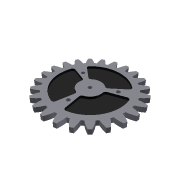
# Autodesk Inventor part: 平歯車1
Saved by Autodesk Inventor 2011 SP1 (Build 150282100, 282)
## iProperties
Created: 2012-11-22
Part Number: 平歯車1
Material: Steel
Document SubType Name: Modeling
Designer: arihon
Categories: <?xml version="1.0" encoding="UTF-16"?> <MemberInstance><Categories><FamilyTemplate><FamilyTemplateParameter ValueType="xs:double" Id="1" ObjectReferenceKey="da_z" ObjectType="kUserParameterObject"/><FamilyTemplateParameter ValueType="xs:double" Id="2" ObjectReferenceKey="da_b" ObjectType="kUserParameterObject"/><FamilyTemplateParameter ValueType="xs:double" Id="3" ObjectReferenceKey="da_beta" ObjectType="kUserParameterObject"/><FamilyTemplateParameter ValueType="xs:double" Id="4" ObjectReferenceKey="da_da" ObjectType="kUserParameterObject"/><FamilyTemplateParameter ValueType="xs:double" Id="5" ObjectReferenceKey="da_aw" ObjectType="kUserParameterObject"/><FamilyTemplateParameter ValueType="xs:string" Id="6" ObjectReferenceKey="EAIAABAAAACIAQAAAAAAAIAAAAAAAAAA" ObjectType="83910656" SubObjectId="SurfaceGeometry"/></FamilyTemplate><ParamToTemplateMap><ParamToTemplate CategoryParameter="//CategoryParameter[@InternalName='046C89C9-8512-4d59-83FE-43B91F4F132A']" TemplateParameter="1"/><ParamToTemplate CategoryParameter="//CategoryParameter[@InternalName='2552DF32-E462-4b46-AEBF-C6C7768E72AC']" TemplateParameter="2"/><ParamToTemplate CategoryParameter="//CategoryParameter[@InternalName='C9EE641D-15FC-4fae-A226-E94C4372FDD7']" TemplateParameter="3"/><ParamToTemplate><ParamToTemplate CategoryParameter="//CategoryParameter[@InternalName='00B6519A-459B-49c7-AD84-2E56D39A5744']" ConstantValue="0.000000"/></ParamToTemplate><ParamToTemplate><ParamToTemplate CategoryParameter="//CategoryParameter[@InternalName='04B31F0E-C7A6-4894-AA32-9629BEFACF47']" ConstantValue="1.000000"/></ParamToTemplate><ParamToTemplate><ParamToTemplate CategoryParameter="//CategoryParameter[@InternalName='43CBEC2E-7847-49e7-A936-2F7889FCB2D9']" ConstantValue="0.250000"/></ParamToTemplate><ParamToTemplate><ParamToTemplate CategoryParameter="//CategoryParameter[@InternalName='B1EFC894-105D-4ebd-86BF-FA20ED196853']" ConstantValue="0.350000"/></ParamToTemplate><ParamToTemplate><ParamToTemplate CategoryParameter="//CategoryParameter[@InternalName='51175063-3D10-4879-93E8-6246FE8B403D']" ConstantValue="2060000000.000000"/></ParamToTemplate><ParamToTemplate><ParamToTemplate CategoryParameter="//CategoryParameter[@InternalName='A3A52E27-4454-46a9-B0BD-C932399B70AF']" ConstantValue="0.300000"/></ParamToTemplate><ParamToTemplate><ParamToTemplate CategoryParameter="//CategoryParameter[@InternalName='91B76062-C214-41d9-B1B9-14D2AB99603D']" ConstantValue="0.300000"/></ParamToTemplate><ParamToTemplate><ParamToTemplate CategoryParameter="//CategoryParameter[@InternalName='374E806E-8B8A-4dda-A9AA-1039D6500AD2']" ConstantValue="3.333333"/></ParamToTemplate><ParamToTemplate><ParamToTemplate CategoryParameter="//CategoryParameter[@InternalName='2D373A89-B862-43d6-8D0B-0CBF12AB9F6C']" ConstantValue="0.349066"/></ParamToTemplate><ParamToTemplate CategoryParameter="//CategoryParameter[@InternalName='37777632-D6A2-4fac-9D53-DB8ACD95C989']" TemplateParameter="4"/><ParamToTemplate CategoryParameter="//CategoryParameter[@InternalName='FD1017F1-B727-4f7e-9707-0F86F1FF9423']" TemplateParameter="5"/><ParamToTemplate><ParamToTemplate CategoryParameter="//CategoryParameter[@InternalName='9E1B4470-B2D3-4ff1-B813-535BB4CDF51A']" ConstantValue="3520000.000000"/></ParamToTemplate><ParamToTemplate><ParamToTemplate CategoryParameter="//CategoryParameter[@InternalName='F8452263-BFF6-458c-9FB1-07C4B99E95CD']" ConstantValue="11400000.000000"/></ParamToTemplate><ParamToTemplate><ParamToTemplate CategoryParameter="//CategoryParameter[@InternalName='3E3BB259-FD49-497f-8171-6EBC954A3479']" ConstantValue="2.000000"/></ParamToTemplate><ParamToTemplate CategoryParameter="//CategoryParameter[@InternalName='27C3BAF2-7550-4e4b-AE2C-0DB134B7D9B7']" TemplateParameter="6"/></ParamToTemplateMap><Category DisplayName="Gear" InternalName="DC85795E-93AB-48d5-8EEE-5A27447B64BD" Mnemonic="Gear"><CategoryParameter DisplayName="z" InternalName="046C89C9-8512-4d59-83FE-43B91F4F132A" Mnemonic="z"/><CategoryParameter DisplayName="b" InternalName="2552DF32-E462-4b46-AEBF-C6C7768E72AC" Mnemonic="b"/><CategoryParameter DisplayName="||b|" InternalName="C9EE641D-15FC-4fae-A226-E94C4372FDD7" Mnemonic="beta"/><CategoryParameter DisplayName="x" InternalName="00B6519A-459B-49c7-AD84-2E56D39A5744" Mnemonic="x"/><CategoryParameter DisplayName="a*" InternalName="04B31F0E-C7A6-4894-AA32-9629BEFACF47" Mnemonic="a"/><CategoryParameter DisplayName="c*" InternalName="43CBEC2E-7847-49e7-A936-2F7889FCB2D9" Mnemonic="c"/><CategoryParameter DisplayName="r|.f|*" InternalName="B1EFC894-105D-4ebd-86BF-FA20ED196853" Mnemonic="rf"/><CategoryParameter DisplayName="E" InternalName="51175063-3D10-4879-93E8-6246FE8B403D" Mnemonic="E"/><CategoryParameter DisplayName="||m|" InternalName="A3A52E27-4454-46a9-B0BD-C932399B70AF" Mnemonic="mi"/><Category DisplayName="SpurGear" InternalName="26C5A22E-A91E-4dfd-A3B3-23CCAFAE1764" Mnemonic="SpurGear"><CategoryParameter DisplayName="m" InternalName="91B76062-C214-41d9-B1B9-14D2AB99603D" Mnemonic="m"/><CategoryParameter DisplayName="P" InternalName="374E806E-8B8A-4dda-A9AA-1039D6500AD2" Mnemonic="PP"/><CategoryParameter DisplayName="||a|" InternalName="2D373A89-B862-43d6-8D0B-0CBF12AB9F6C" Mnemonic="alpha"/><CategoryParameter DisplayName="d|.a|" InternalName="37777632-D6A2-4fac-9D53-DB8ACD95C989" Mnemonic="da"/><CategoryParameter DisplayName="a|.w|" InternalName="FD1017F1-B727-4f7e-9707-0F86F1FF9423" Mnemonic="aw"/><CategoryParameter DisplayName="||s||.Flim|" InternalName="9E1B4470-B2D3-4ff1-B813-535BB4CDF51A" Mnemonic="sFlim"/><CategoryParameter DisplayName="||s||.Hlim|" InternalName="F8452263-BFF6-458c-9FB1-07C4B99E95CD" Mnemonic="sHlim"/><CategoryParameter DisplayName="種類" InternalName="3E3BB259-FD49-497f-8171-6EBC954A3479" Mnemonic="type"/><CategoryParameter DisplayName="PitchDiameter" InternalName="27C3BAF2-7550-4e4b-AE2C-0DB134B7D9B7" Mnemonic="IDS_PITCHDIAM"/></Category></Category></Categories></MemberInstance>
Density: 1 g/cm^3
CustomPartVersion: 1
Author: arihon
Autodesk Inventor part; units mm, degrees
ref_plane "YZ Plane" through (0, 0, 0) normal (1, 0, 0) x (0, 1, 0)
ref_plane "XZ Plane" through (0, 0, 0) normal (0, 1, 0) x (-1, 0, 0)
ref_plane "XY Plane" through (0, 0, 0) normal (0, 0, 1) x (1, 0, 0)
sketch "Sketch1" plane through (0, 0, 0) normal (0, 0, 1) x (1, 0, 0)
  circle A0 centre (0, 0) radius 38.9632
  dimension "d0" = 77.9263
  constraints: 1 centre point
  measures "d0" diameter of A0
extrude "Extrusion1" add sketch "Sketch1" along normal blind 5
ref_plane "Work Plane2" through (0, 0, 2.5) normal (0, 0, 1) x (1, 0, 0)
sketch "Sketch2" plane through (0, 0, 0) normal (0, 0, -1) x (-1, 0, 0)
  circle A0 centre (0, 0) radius 38.9632 projected
  circle A1 centre (0, 0) radius 36.3636
  dimension "d3" = 72.7273
  constraints: 1 centre point, 1 coincident
  measures "d3" diameter of A1
surface extrude "ピッチ円直径" sketch "Sketch2" against normal through all shown no curves A1
ref_plane "Work Plane8" through (0, 0, 0) normal (0.9914449, 0.1305262, 0) x (0, 0, 1)
ref_plane "Work Plane9" through (0, 0, 0) normal (1, 0, 0) x (0, 1, 0)
spur gear teeth "平歯車" teeth 24 pitch diameter 72 tip diameter 77.9263 root diameter 64.5 face width 5 start plane through (0, 0, 0) normal (0, 0, -1) x (-1, 0, 0)
sketch "スケッチ3" plane through (0, 0, 5) normal (0, 0, 1) x (1, 0, 0)
  arc A0 (-8.8476, 37.9453) -> (-11.3104, 37.2854) centre (0, 0) ccw projected
  arc A1 (-21.0662, 17.6767) -> (21.0662, 17.6767) centre (0, 0) ccw
  arc A2 (0, 10) -> (-7.6604, 6.4279) centre (0, 0) ccw
  line L0 (0, 0) -> (-7.6604, 6.4279)
  line L1 (0, 0) -> (7.6604, 6.4279)
  line L2 (0, 0) -> (0, 27.5)
  line L3 (7.6604, 6.4279) -> (21.0662, 17.6767)
  line L4 (-7.6604, 6.4279) -> (-21.0662, 17.6767)
  arc A3 (0, 27.5) -> (-21.0662, 17.6767) centre (0, 0) ccw
  arc A4 (21.0662, 17.6767) -> (0, 27.5) centre (0, 0) ccw
  arc A5 (7.6604, 6.4279) -> (0, 10) centre (0, 0) ccw
  arc A6 (-7.6604, 6.4279) -> (7.6604, 6.4279) centre (0, 0) ccw
  dimension "d49" = 55
  dimension "d50" = 20
  dimension "d51" = 100
  dimension "d52" = 50
  constraints: 12 point on circle, 10 end point, 6 centre point, 3 coincident, 1 point on line, 1 vertical
  measures "d49" diameter of A1
  measures "d50" diameter of A2
  measures "d51" angle of L1 L0
  measures "d52" angle of L1 L2
extrude "押し出し2" cut sketch "スケッチ3" against normal blind 3 contours A3 L2 A2 L4 | L3 A5 L2 A4
fillet "フィレット1" radius 2 4 edges at (-21.0662, 17.6767, 3.5) (-7.6604, 6.4279, 3.5) (7.6604, 6.4279, 3.5) (21.0662, 17.6767, 3.5)
pattern_circular "放射状パターン1" count 3 over 360 about axis through (0, 0, 5) along (0, 0, -1) of "押し出し2", "フィレット1"
sketch "スケッチ5" plane through (0, 0, 5) normal (0, 0, 1) x (1, 0, 0)
  line L0 (19.474, 16.3406) -> (9.064, 7.6056) projected
  arc A0 (20.5752, 33.0876) -> (18.3671, 34.3624) centre (0, 0) ccw projected
  arc A1 (-8.8476, 37.9453) -> (-11.3104, 37.2854) centre (0, 0) ccw projected
  circle A2 centre (0, 0) radius 18.75
  line L1 (0, 0) -> (0, 18.75)
  line L2 (0, 0) -> (16.238, 9.375)
  point P0 (16.238, 9.375)
  point P1 (-16.238, 9.375)
  point P2 (0, -18.75)
  dimension "d71" = 37.5
  dimension "d72" = 60
  dimension "d75" = 360
  constraints: 4 end point, 3 coincident, 2 point on circle, 1 centre point, 1 point on line, 1 vertical, 4 other
  measures "d71" diameter of A2
  measures "d72" angle of L2 L1
hole "Hole2" at (16.238, 9.375, 5) at (-16.238, 9.375, 5) at (0, -18.75, 5) at (0, 0, 5) direction (0, 0, -1) diameter 3.2 depth 8 tip angle 118
sketch "スケッチ6" plane through (0, 0, 5) normal (0, 0, 1) x (1, 0, 0)
  circle A0 centre (0, 0) radius 1.6 projected
  circle A1 centre (0, -18.75) radius 1.6 projected
  circle A2 centre (-16.238, 9.375) radius 1.6 projected
  circle A3 centre (16.238, 9.375) radius 1.6 projected
  line L0 (-23.8883, 8.6946) -> (-11.1186, 4.0468) projected
  arc A4 (-9.8355, 1.8062) -> (-11.1186, 4.0468) centre (-11.8026, 2.1675) ccw projected
  arc A5 (-9.8355, 1.8062) -> (-3.3535, -9.4209) centre (0, 0) ccw projected
  arc A6 (-2.0546, -11.6524) -> (-3.3535, -9.4209) centre (-4.0242, -11.3051) ccw projected
  line L1 (-2.0546, -11.6524) -> (-4.4144, -25.0352) projected
  arc A7 (-6.8847, -26.6243) -> (-4.4144, -25.0352) centre (-6.384, -24.6879) ccw projected
  arc A8 (-26.4996, 7.3498) -> (-6.8847, -26.6243) centre (0, 0) ccw projected
  arc A9 (-23.8883, 8.6946) -> (-26.4996, 7.3498) centre (-24.5724, 6.8153) ccw projected
  line L2 (4.4144, -25.0352) -> (2.0546, -11.6524) projected
  arc A10 (3.3535, -9.4209) -> (2.0546, -11.6524) centre (4.0242, -11.3051) ccw projected
  arc A11 (3.3535, -9.4209) -> (9.8355, 1.8062) centre (0, 0) ccw projected
  arc A12 (11.1186, 4.0468) -> (9.8355, 1.8062) centre (11.8026, 2.1675) ccw projected
  line L3 (11.1186, 4.0468) -> (23.8883, 8.6946) projected
  arc A13 (26.4996, 7.3498) -> (23.8883, 8.6946) centre (24.5724, 6.8153) ccw projected
  arc A14 (6.8847, -26.6243) -> (26.4996, 7.3498) centre (0, 0) ccw projected
  arc A15 (4.4144, -25.0352) -> (6.8847, -26.6243) centre (6.384, -24.6879) ccw projected
  line L4 (19.474, 16.3406) -> (9.064, 7.6056) projected
  arc A16 (6.482, 7.6147) -> (9.064, 7.6056) centre (7.7784, 9.1377) ccw projected
  arc A17 (6.482, 7.6147) -> (-6.482, 7.6147) centre (0, 0) ccw projected
  arc A18 (-9.064, 7.6056) -> (-6.482, 7.6147) centre (-7.7784, 9.1377) ccw projected
  line L5 (-9.064, 7.6056) -> (-19.474, 16.3406) projected
  arc A19 (-19.6149, 19.2745) -> (-19.474, 16.3406) centre (-18.1884, 17.8727) ccw projected
  arc A20 (19.6149, 19.2745) -> (-19.6149, 19.2745) centre (0, 0) ccw projected
  arc A21 (19.474, 16.3406) -> (19.6149, 19.2745) centre (18.1884, 17.8727) ccw projected
  arc A22 (-11.3104, 37.2854) -> (-11.3601, 30.183) centre (15.4473, 33.5469) ccw projected
  arc A23 (-11.3601, 30.183) -> (-13.3098, 29.3754) centre (0, 0) ccw projected
  arc A24 (-13.3098, 29.3754) -> (-18.3671, 34.3624) centre (-34.6442, 12.7984) ccw projected
  arc A25 (-18.3671, 34.3624) -> (-20.5752, 33.0876) centre (0, 0) ccw projected
  arc A26 (-20.5752, 33.0876) -> (-18.7849, 26.2143) centre (6.2384, 36.4019) ccw projected
  arc A27 (-18.7849, 26.2143) -> (-20.4592, 24.9296) centre (0, 0) ccw projected
  arc A28 (-20.4592, 24.9296) -> (-26.6349, 28.4378) centre (-36.7762, 3.3957) ccw projected
  arc A29 (-26.6349, 28.4378) -> (-28.4378, 26.6349) centre (0, 0) ccw projected
  arc A30 (-28.4378, 26.6349) -> (-24.9296, 20.4592) centre (-3.3957, 36.7762) ccw projected
  arc A31 (-24.9296, 20.4592) -> (-26.2143, 18.7849) centre (0, 0) ccw projected
  arc A32 (-26.2143, 18.7849) -> (-33.0876, 20.5752) centre (-36.4019, -6.2384) ccw projected
  arc A33 (-33.0876, 20.5752) -> (-34.3624, 18.3671) centre (0, 0) ccw projected
  arc A34 (-34.3624, 18.3671) -> (-29.3754, 13.3098) centre (-12.7984, 34.6442) ccw projected
  arc A35 (-29.3754, 13.3098) -> (-30.183, 11.3601) centre (0, 0) ccw projected
  arc A36 (-30.183, 11.3601) -> (-37.2854, 11.3104) centre (-33.5469, -15.4473) ccw projected
  arc A37 (-37.2854, 11.3104) -> (-37.9453, 8.8476) centre (0, 0) ccw projected
  arc A38 (-37.9453, 8.8476) -> (-31.8192, 5.2534) centre (-21.3288, 30.1512) ccw projected
  arc A39 (-31.8192, 5.2534) -> (-32.0947, 3.1611) centre (0, 0) ccw projected
  arc A40 (-32.0947, 3.1611) -> (-38.9423, 1.2748) centre (-28.4058, -23.6035) ccw projected
  arc A41 (-38.9423, 1.2748) -> (-38.9423, -1.2748) centre (0, 0) ccw projected
  arc A42 (-38.9423, -1.2748) -> (-32.0947, -3.1611) centre (-28.4058, 23.6035) ccw projected
  arc A43 (-32.0947, -3.1611) -> (-31.8192, -5.2534) centre (0, 0) ccw projected
  arc A44 (-31.8192, -5.2534) -> (-37.9453, -8.8476) centre (-21.3288, -30.1512) ccw projected
  arc A45 (-37.9453, -8.8476) -> (-37.2854, -11.3104) centre (0, 0) ccw projected
  arc A46 (-37.2854, -11.3104) -> (-30.183, -11.3601) centre (-33.5469, 15.4473) ccw projected
  arc A47 (-30.183, -11.3601) -> (-29.3754, -13.3098) centre (0, 0) ccw projected
  arc A48 (-29.3754, -13.3098) -> (-34.3624, -18.3671) centre (-12.7984, -34.6442) ccw projected
  arc A49 (-34.3624, -18.3671) -> (-33.0876, -20.5752) centre (0, 0) ccw projected
  arc A50 (-33.0876, -20.5752) -> (-26.2143, -18.7849) centre (-36.4019, 6.2384) ccw projected
  arc A51 (-26.2143, -18.7849) -> (-24.9296, -20.4592) centre (0, 0) ccw projected
  arc A52 (-24.9296, -20.4592) -> (-28.4378, -26.6349) centre (-3.3957, -36.7762) ccw projected
  arc A53 (-28.4378, -26.6349) -> (-26.6349, -28.4378) centre (0, 0) ccw projected
  arc A54 (-26.6349, -28.4378) -> (-20.4592, -24.9296) centre (-36.7762, -3.3957) ccw projected
  arc A55 (-20.4592, -24.9296) -> (-18.7849, -26.2143) centre (0, 0) ccw projected
  arc A56 (-18.7849, -26.2143) -> (-20.5752, -33.0876) centre (6.2384, -36.4019) ccw projected
  arc A57 (-20.5752, -33.0876) -> (-18.3671, -34.3624) centre (0, 0) ccw projected
  arc A58 (-18.3671, -34.3624) -> (-13.3098, -29.3754) centre (-34.6442, -12.7984) ccw projected
  arc A59 (-13.3098, -29.3754) -> (-11.3601, -30.183) centre (0, 0) ccw projected
  arc A60 (-11.3601, -30.183) -> (-11.3104, -37.2854) centre (15.4473, -33.5469) ccw projected
  arc A61 (-11.3104, -37.2854) -> (-8.8476, -37.9453) centre (0, 0) ccw projected
  arc A62 (-8.8476, -37.9453) -> (-5.2534, -31.8192) centre (-30.1512, -21.3288) ccw projected
  arc A63 (-5.2534, -31.8192) -> (-3.1611, -32.0947) centre (0, 0) ccw projected
  arc A64 (-3.1611, -32.0947) -> (-1.2748, -38.9423) centre (23.6035, -28.4058) ccw projected
  arc A65 (-1.2748, -38.9423) -> (1.2748, -38.9423) centre (0, 0) ccw projected
  arc A66 (1.2748, -38.9423) -> (3.1611, -32.0947) centre (-23.6035, -28.4058) ccw projected
  arc A67 (3.1611, -32.0947) -> (5.2534, -31.8192) centre (0, 0) ccw projected
  arc A68 (5.2534, -31.8192) -> (8.8476, -37.9453) centre (30.1512, -21.3288) ccw projected
  arc A69 (8.8476, -37.9453) -> (11.3104, -37.2854) centre (0, 0) ccw projected
  arc A70 (11.3104, -37.2854) -> (11.3601, -30.183) centre (-15.4473, -33.5469) ccw projected
  arc A71 (11.3601, -30.183) -> (13.3098, -29.3754) centre (0, 0) ccw projected
  arc A72 (13.3098, -29.3754) -> (18.3671, -34.3624) centre (34.6442, -12.7984) ccw projected
  arc A73 (18.3671, -34.3624) -> (20.5752, -33.0876) centre (0, 0) ccw projected
  arc A74 (20.5752, -33.0876) -> (18.7849, -26.2143) centre (-6.2384, -36.4019) ccw projected
  arc A75 (18.7849, -26.2143) -> (20.4592, -24.9296) centre (0, 0) ccw projected
  arc A76 (20.4592, -24.9296) -> (26.6349, -28.4378) centre (36.7762, -3.3957) ccw projected
  arc A77 (26.6349, -28.4378) -> (28.4378, -26.6349) centre (0, 0) ccw projected
  arc A78 (28.4378, -26.6349) -> (24.9296, -20.4592) centre (3.3957, -36.7762) ccw projected
  arc A79 (24.9296, -20.4592) -> (26.2143, -18.7849) centre (0, 0) ccw projected
  arc A80 (26.2143, -18.7849) -> (33.0876, -20.5752) centre (36.4019, 6.2384) ccw projected
  arc A81 (33.0876, -20.5752) -> (34.3624, -18.3671) centre (0, 0) ccw projected
  arc A82 (34.3624, -18.3671) -> (29.3754, -13.3098) centre (12.7984, -34.6442) ccw projected
  arc A83 (29.3754, -13.3098) -> (30.183, -11.3601) centre (0, 0) ccw projected
  arc A84 (30.183, -11.3601) -> (37.2854, -11.3104) centre (33.5469, 15.4473) ccw projected
  arc A85 (37.2854, -11.3104) -> (37.9453, -8.8476) centre (0, 0) ccw projected
  arc A86 (37.9453, -8.8476) -> (31.8192, -5.2534) centre (21.3288, -30.1512) ccw projected
  arc A87 (31.8192, -5.2534) -> (32.0947, -3.1611) centre (0, 0) ccw projected
  arc A88 (32.0947, -3.1611) -> (38.9423, -1.2748) centre (28.4058, 23.6035) ccw projected
  arc A89 (38.9423, -1.2748) -> (38.9423, 1.2748) centre (0, 0) ccw projected
  arc A90 (38.9423, 1.2748) -> (32.0947, 3.1611) centre (28.4058, -23.6035) ccw projected
  arc A91 (32.0947, 3.1611) -> (31.8192, 5.2534) centre (0, 0) ccw projected
  arc A92 (31.8192, 5.2534) -> (37.9453, 8.8476) centre (21.3288, 30.1512) ccw projected
  arc A93 (37.9453, 8.8476) -> (37.2854, 11.3104) centre (0, 0) ccw projected
  arc A94 (37.2854, 11.3104) -> (30.183, 11.3601) centre (33.5469, -15.4473) ccw projected
  arc A95 (30.183, 11.3601) -> (29.3754, 13.3098) centre (0, 0) ccw projected
  arc A96 (29.3754, 13.3098) -> (34.3624, 18.3671) centre (12.7984, 34.6442) ccw projected
  arc A97 (34.3624, 18.3671) -> (33.0876, 20.5752) centre (0, 0) ccw projected
  arc A98 (33.0876, 20.5752) -> (26.2143, 18.7849) centre (36.4019, -6.2384) ccw projected
  arc A99 (26.2143, 18.7849) -> (24.9296, 20.4592) centre (0, 0) ccw projected
  arc A100 (24.9296, 20.4592) -> (28.4378, 26.6349) centre (3.3957, 36.7762) ccw projected
  arc A101 (28.4378, 26.6349) -> (26.6349, 28.4378) centre (0, 0) ccw projected
  arc A102 (26.6349, 28.4378) -> (20.4592, 24.9296) centre (36.7762, 3.3957) ccw projected
  arc A103 (20.4592, 24.9296) -> (18.7849, 26.2143) centre (0, 0) ccw projected
  arc A104 (18.7849, 26.2143) -> (20.5752, 33.0876) centre (-6.2384, 36.4019) ccw projected
  arc A105 (20.5752, 33.0876) -> (18.3671, 34.3624) centre (0, 0) ccw projected
  arc A106 (18.3671, 34.3624) -> (13.3098, 29.3754) centre (34.6442, 12.7984) ccw projected
  arc A107 (13.3098, 29.3754) -> (11.3601, 30.183) centre (0, 0) ccw projected
  arc A108 (11.3601, 30.183) -> (11.3104, 37.2854) centre (-15.4473, 33.5469) ccw projected
  arc A109 (11.3104, 37.2854) -> (8.8476, 37.9453) centre (0, 0) ccw projected
  arc A110 (8.8476, 37.9453) -> (5.2534, 31.8192) centre (30.1512, 21.3288) ccw projected
  arc A111 (5.2534, 31.8192) -> (3.1611, 32.0947) centre (0, 0) ccw projected
  arc A112 (3.1611, 32.0947) -> (1.2748, 38.9423) centre (-23.6035, 28.4058) ccw projected
  arc A113 (1.2748, 38.9423) -> (-1.2748, 38.9423) centre (0, 0) ccw projected
  arc A114 (-1.2748, 38.9423) -> (-3.1611, 32.0947) centre (23.6035, 28.4058) ccw projected
  arc A115 (-3.1611, 32.0947) -> (-5.2534, 31.8192) centre (0, 0) ccw projected
  arc A116 (-5.2534, 31.8192) -> (-8.8476, 37.9453) centre (-30.1512, 21.3288) ccw projected
  arc A117 (-8.8476, 37.9453) -> (-11.3104, 37.2854) centre (0, 0) ccw projected
extrude "押し出し3" cut sketch "スケッチ6" against normal blind 1
equation "\"d0\" = da_da"
equation "\"d1\" = da_b"
equation "\"d3\" = da_dw"
equation "\"d52\" = 0.5 * d51"
equation "\"da_da\" = 77.926309"
equation "\"da_b\" = 5"
equation "\"da_dw\" = 72.727273"
body "Solid1"
body "Srf1"
